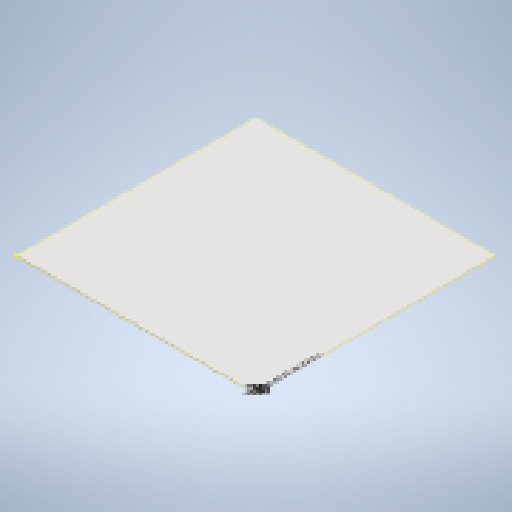
# Autodesk Inventor part: testbase
Saved by Autodesk Inventor 2025 (Build 290162000, 162)
## iProperties
Created: 2025-05-11
Part Number: testbase
Material: Generic
Document SubType Name: Modeling
Designer: ethan
Density: 1 g/cm^3
Appearance: Default
Author: ethan
Autodesk Inventor part; units mm, degrees
ref_plane "YZ Plane" through (0, 0, 0) normal (1, 0, 0) x (0, 1, 0)
ref_plane "XZ Plane" through (0, 0, 0) normal (0, 1, 0) x (-1, 0, 0)
ref_plane "XY Plane" through (0, 0, 0) normal (0, 0, 1) x (1, 0, 0)
sketch "Sketch1" plane through (0, 0, 0) normal (0, 1, 0) x (-1, 0, 0)
  line L0 (0, 0) -> (-152.4, 0)
  line L1 (-152.4, 0) -> (-152.4, -228.6)
  line L2 (-152.4, -228.6) -> (0, -228.6)
  line L3 (0, -228.6) -> (0, 0)
  dimension "d0" = 152.4
  dimension "d1" = 228.6
  constraints: 8 end point, 2 parallel, 1 horizontal, 1 perpendicular
  measures "d0" distance of L2.end L1.end
  measures "d1" distance of L1.end L0.end
extrude "Extrusion1" add sketch "Sketch1" along normal blind 2
sketch "Sketch3" plane through (0, 2, 0) normal (0, 1, 0) x (1, 0, 0)
  line L0 (152.4, 0) -> (152.4, 228.6) projected
  line L1 (152.4, 228.6) -> (0, 228.6) projected
  line L2 (0, 228.6) -> (0, 0) projected
  line L3 (0, 0) -> (152.4, 0) projected
  line L4 (3, 3) -> (3, 225.6)
  line L5 (3, 225.6) -> (149.4, 225.6)
  line L6 (149.4, 225.6) -> (149.4, 3)
  line L7 (149.4, 3) -> (3, 3)
  dimension "d13" = 3
  constraints: 8 end point, 3 other
  measures "d13" distance between parallel lines of L2 L4
extrude "Extrusion2" add sketch "Sketch3" along normal blind 2.54
sketch "Sketch4" plane through (0, 4.54, 0) normal (0, 1, 0) x (1, 0, 0)
  line L0 (152.4, 228.6) -> (0, 228.6) projected
  line L1 (0, 228.6) -> (0, 0) projected
  line L2 (0, 0) -> (152.4, 0) projected
  line L3 (152.4, 0) -> (152.4, 228.6) projected
  line L4 (3, 3) -> (3, 225.6) projected
  line L5 (3, 225.6) -> (149.4, 225.6) projected
  line L6 (149.4, 225.6) -> (149.4, 3) projected
  line L7 (149.4, 3) -> (3, 3) projected
  line L8 (152.4, 225.6) -> (0, 225.6)
  line L9 (0, 225.6) -> (0, 228.6)
  line L10 (0, 228.6) -> (152.4, 228.6)
  line L11 (152.4, 228.6) -> (152.4, 225.6)
  line L12 (0, 0) -> (152.4, 0)
  line L13 (152.4, 0) -> (152.4, 3)
  line L14 (152.4, 3) -> (0, 3)
  line L15 (0, 3) -> (0, 0)
  constraints: 16 end point, 4 parallel, 2 horizontal, 2 perpendicular, 2 point on line
extrude "Extrusion3" add sketch "Sketch4" along normal blind 69.85 separate body contours L3 L8 L5 L1 L0 | L3 L2 L1 L14 L7
body "Solid1"
body "Solid2"
